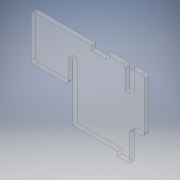
# Autodesk Inventor part: front_right_v2
Saved by Autodesk Inventor 2017.2 (Build 212233000, 233)
## iProperties
Created: 2017-06-09
Part Number: front_right_v2
Material: Generic
Document SubType Name: Modeling
Designer: SandeepSH
Density: 1 g/cm^3
Appearance: Polycarbonate - Clear
Author: SandeepSH
Autodesk Inventor part; units mm, degrees
ref_plane "YZ Plane" through (0, 0, 0) normal (1, 0, 0) x (0, 1, 0)
ref_plane "XZ Plane" through (0, 0, 0) normal (0, 1, 0) x (-1, 0, 0)
ref_plane "XY Plane" through (0, 0, 0) normal (0, 0, 1) x (1, 0, 0)
sketch "Sketch1" plane through (0, 0, 0) normal (0, 0, 1) x (1, 0, 0)
  line L0 (0, 0) -> (41, 0)
  line L1 (41, 0) -> (41, 55.5)
  line L2 (41, 55.5) -> (0, 55.5)
  line L3 (0, 55.5) -> (0, 0)
  dimension "d0" = 41
  dimension "d1" = 55.5
  constraints: 8 end point, 2 parallel, 1 horizontal, 1 perpendicular
  measures "d0" distance of L2.end L1.end
  measures "d1" distance of L1.end L0.end
extrude "Extrusion1" add sketch "Sketch1" along normal blind 3
sketch "Sketch2" plane through (0, 0, 3) normal (0, 0, 1) x (1, 0, 0)
  line L0 (0, 0) -> (33, 0)
  line L1 (33, 0) -> (33, 3)
  line L2 (33, 3) -> (0, 3)
  line L3 (0, 3) -> (0, 0)
  line L4 (41, 0) -> (41, 55.5) projected
  line L5 (0, 3) -> (3, 3)
  line L6 (3, 3) -> (3, 40.5)
  line L7 (3, 40.5) -> (0, 40.5)
  line L8 (0, 40.5) -> (0, 3)
  line L9 (41, 55.5) -> (0, 55.5) projected
  line L10 (15.5, 55.5) -> (25.5, 55.5)
  line L11 (25.5, 55.5) -> (25.5, 52.5)
  line L12 (25.5, 52.5) -> (15.5, 52.5)
  line L13 (15.5, 52.5) -> (15.5, 55.5)
  line L14 (41, 55.5) -> (38, 55.5)
  line L15 (38, 55.5) -> (38, 40.5)
  line L16 (38, 40.5) -> (41, 40.5)
  line L17 (41, 40.5) -> (41, 55.5)
  line L18 (0, 55.5) -> (0, 0) projected
  point P0 (20.5, 52.5)
  dimension "d4" = 3
  dimension "d5" = 8
  dimension "d6" = 3
  dimension "d7" = 15
  dimension "d8" = 10
  dimension "d9" = 3
  dimension "d11" = 3
  dimension "d12" = 15
  dimension "d23" = 41
  dimension "d24" = 20.5
  constraints: 32 end point, 8 parallel, 4 horizontal, 4 perpendicular, 1 midpoint, 1 point on line
  measures "d4" distance of L1.end L0.end
  measures "d5" distance between parallel lines of L4 L1
  measures "d6" distance of L7.end L6.end
  measures "d7" distance between parallel lines of L9 L7
  measures "d8" distance of L11.end L12.end
  measures "d9" distance of L10.end L11.end
  measures "d11" distance of L16.end L15.end
  measures "d12" distance of L15.end L14.end
  measures "d23" distance between parallel lines of L4 L18
  measures "d24" distance from line of L4 point (20.5, 52.5)
extrude "Extrusion2" cut sketch "Sketch2" against normal through all
sketch "Sketch3" plane through (0, 0, 3) normal (0, 0, 1) x (1, 0, 0)
  line L0 (15.5, 55.5) -> (0, 55.5) projected
  line L1 (0, 55.5) -> (-25, 55.5)
  line L2 (-25, 55.5) -> (-25, 25)
  line L3 (-25, 25) -> (0, 25)
  line L4 (0, 25) -> (0, 55.5)
  line L5 (33, 0) -> (41, 0) projected
  line L6 (41, 55.5) -> (51, 55.5)
  line L7 (51, 55.5) -> (51, 20)
  line L8 (51, 20) -> (41, 20)
  line L9 (41, 20) -> (41, 55.5)
  line L10 (38, 55.5) -> (25.5, 55.5) projected
  line L11 (41, 0) -> (41, 40.5) projected
  point P0 (0, 0)
  dimension "d15" = 25
  dimension "d16" = 25
  dimension "d17" = 10
  dimension "d18" = 20
  constraints: 16 end point, 4 parallel, 2 collinear, 2 horizontal, 2 perpendicular
  measures "d15" distance of L3.end L2.end
  measures "d16" distance between parallel lines of L5 L3
  measures "d17" distance of L7.end L8.end
  measures "d18" distance between parallel lines of L5 L8
extrude "Extrusion3" add sketch "Sketch3" against normal blind 3
fillet "Fillet1" radius 2 7 edges at (0, 25, 1.5) (51, 20, 1.5) (51, 55.5, 1.5) (38, 55.5, 1.5) (41, 55.5, 1.5) (41, 20, 1.5) (-25, 25, 1.5) curvature continuous yes
fillet "Fillet2" radius 2 1 edges at (-25, 55.5, 1.5) curvature continuous yes
equation "\"d24\" = 0.5 * d23"
body "Solid1"
